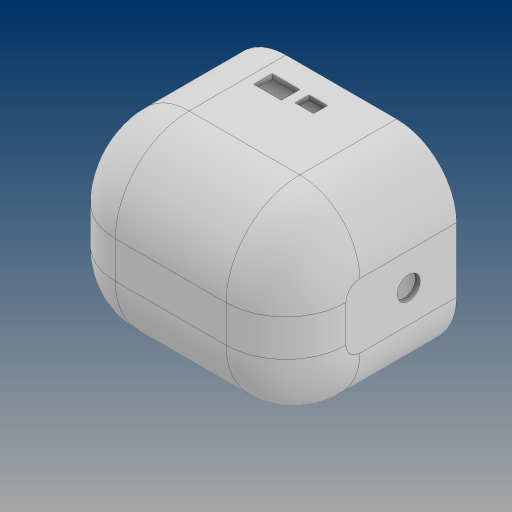
# Autodesk Inventor part: Protosaber Case
Saved by Autodesk Inventor 2023 (Build 270158000, 158)
## iProperties
Created: 2023-05-22
Part Number: Protosaber Case
Material: Generic
Document SubType Name: Modeling
Designer: joosv
Density: 1 g/cm^3
Appearance: Default
Author: joosv
Autodesk Inventor part; units mm, degrees
ref_plane "YZ Plane" through (0, 0, 0) normal (1, 0, 0) x (0, 1, 0)
ref_plane "XZ Plane" through (0, 0, 0) normal (0, 1, 0) x (-1, 0, 0)
ref_plane "XY Plane" through (0, 0, 0) normal (0, 0, 1) x (1, 0, 0)
sketch "Sketch1" plane through (0, 0, 0) normal (0, 0, 1) x (1, 0, 0)
  line L0 (-175, 0) -> (175, 0) projected
  line L1 (0, -140) -> (0, 140) projected
  line L2 (-125, 100) -> (125, 100)
  line L3 (125, 100) -> (125, -100)
  line L4 (125, -100) -> (-125, -100)
  line L5 (-125, -100) -> (-125, 100)
  point P0 (0, 0)
  dimension "d0" = 200
  dimension "d1" = 250
  constraints: 8 end point, 2 parallel, 1 horizontal, 1 perpendicular, 2 other
  measures "d0" distance of L4.end L2.start
  measures "d1" distance of L2.start L2.end
extrude "Extrusion1" add sketch "Sketch1" against normal blind 180
fillet "Fillet5" radius 80 2 edges at (0, -100, 0) (0, 100, 0)
fillet "Fillet6" radius 65 10 edges at (125, 0, 0) (125, 76.5685, -23.4315) (125, 100, -130) (125, -100, -130) (125, -76.5685, -23.4315) (-125, -100, -130) (-125, 0, 0) (-125, 76.5685, -23.4315) (-125, 100, -130) (-125, -76.5685, -23.4315)
shell "Shell1" thickness 5 removed faces 1 at (20, -33.3333, -180)
sketch "Sketch5" plane through (-60, -100, -180) normal (0, -1, 0) x (1, 0, 0)
  line L0 (120, 0) -> (120, 100) projected
  line L1 (70, 96.5308) -> (120, 96.5308)
  line L2 (120, 96.5308) -> (120, 71.5308)
  line L3 (120, 71.5308) -> (70, 71.5308)
  line L4 (70, 71.5308) -> (70, 96.5308)
  point P0 (60, 180)
  dimension "d15" = 25
  dimension "d16" = 50
  constraints: 8 end point, 2 parallel, 1 horizontal, 1 perpendicular, 1 point on line
  measures "d15" distance between parallel lines of L3 L1
  measures "d16" distance between parallel lines of L0 L4
extrude "Extrusion3" cut sketch "Sketch5" against normal blind 24
sketch "Sketch6" plane through (-60, -100, -80) normal (0, -1, 0) x (1, 0, 0)
  circle A0 centre (55, -15.7839) radius 7.5
  line L0 (70, -28.4692) -> (70, -3.4692) projected
  point P0 (60, 80)
  point P1 (70, -15.9692)
  dimension "d19" = 15
  dimension "d20" = 15
  constraints: 1 centre point, 1 midpoint
  measures "d19" diameter of A0
  measures "d20" horizontal distance of point (70, -15.969) A0.centre
extrude "Extrusion4" add sketch "Sketch6" along normal blind 25
sketch "Sketch7" plane through (-60, -100, -80) normal (0, -1, 0) x (1, 0, 0)
  circle A0 centre (95, -60.7349) radius 11
  line L0 (120, -28.4692) -> (120, -100) projected
  point P0 (60, 80)
  dimension "d23" = 25
  dimension "d24" = 22
  constraints: 1 centre point
  measures "d23" distance from line of L0 A0.centre
  measures "d24" diameter of A0
extrude "Extrusion5" add sketch "Sketch7" along normal blind 20
fillet "Fillet7" radius 1.5 1 edges at (-12.5, -125, -95.7839)
fillet "Fillet8" radius 1.5 1 edges at (24, -120, -140.7349)
sketch "Sketch8" plane through (-60, -95, -180) normal (0, 1, 0) x (1, 0, 0)
  line L0 (120, -96.5308) -> (70, -96.5308) projected
  line L1 (70, -96.5308) -> (70, -71.5308) projected
  line L2 (70, -71.5308) -> (120, -71.5308) projected
  line L3 (120, -71.5308) -> (120, 0) projected
  line L4 (0, 0) -> (120, 0) projected
  line L5 (0, 0) -> (0, -100) projected
  line L6 (0, -100) -> (120, -100) projected
  line L7 (120, -100) -> (120, -96.5308) projected
  line L8 (103.331, -9.0858) -> (93.331, -9.0858)
  line L9 (93.331, -9.0858) -> (93.331, -12.0858)
  line L10 (93.331, -12.0858) -> (103.331, -12.0858)
  line L11 (103.331, -12.0858) -> (103.331, -9.0858)
  line L12 (60, -9.0858) -> (50, -9.0858)
  line L13 (50, -9.0858) -> (50, -12.0858)
  line L14 (50, -12.0858) -> (60, -12.0858)
  line L15 (60, -12.0858) -> (60, -9.0858)
  point P0 (60, -180)
  dimension "d29" = 10
  dimension "d30" = 3
  dimension "d31" = 10
  constraints: 16 end point, 4 parallel, 2 horizontal, 2 perpendicular, 2 point on line
  measures "d29" distance of L10.end L9.end
  measures "d30" distance of L9.end L8.end
  measures "d31" distance of L14.end L13.end
extrude "Extrusion6" add sketch "Sketch8" along normal blind 15 contours L11 L10 L9 L8 | L15 L14 L13 L12
sketch "Sketch9" plane through (-10, -95, -167.9142) normal (0, 0, 1) x (1, 0, 0)
  line L0 (0, 0) -> (0, 15) projected
  line L1 (10, 0) -> (10, 15) projected
  line L2 (0, 9.5743) -> (10, 9.5743)
  line L3 (10, 9.5743) -> (10, 15)
  line L4 (10, 15) -> (0, 15)
  line L5 (0, 15) -> (0, 9.5743)
  line L6 (53.331, 15) -> (43.331, 15) projected
  line L7 (43.2725, 9.5743) -> (53.331, 9.5743)
  line L8 (53.331, 9.5743) -> (53.331, 15)
  line L9 (53.331, 15) -> (43.2725, 15)
  line L10 (43.2725, 15) -> (43.2725, 9.5743)
  point P0 (10, 95)
  constraints: 16 end point, 4 parallel, 2 horizontal, 2 perpendicular, 2 point on line
extrude "Extrusion7" add sketch "Sketch9" along normal blind 5
sketch "Sketch10" plane through (125, -35, -180) normal (1, 0, 0) x (0, 0, -1)
  line L0 (0, 0) -> (-100, 0) projected
  line L1 (0, 70) -> (0, 0) projected
  line L2 (-100, 70) -> (0, 70) projected
  arc A0 (-100, 70) -> (-115, 55) centre (-100, 55) ccw projected
  line L3 (-115, 15) -> (-115, 55) projected
  arc A1 (-115, 15) -> (-100, 0) centre (-100, 15) ccw projected
  circle A2 centre (-47.024, 35) radius 12.5
  point P0 (-180, 35)
  dimension "d36" = 25
  constraints: 1 centre point
  measures "d36" diameter of A2
extrude "Extrusion8" cut sketch "Sketch10" against normal blind 25 contours A2
sketch "Sketch11" plane through (-60, 100, -80) normal (0, 1, 0) x (1, 0, 0)
  line L0 (40, 60) -> (10, 60)
  line L1 (10, 60) -> (10, 80)
  line L2 (10, 80) -> (40, 80)
  line L3 (40, 80) -> (40, 60)
  line L4 (0, 0) -> (0, 100) projected
  line L5 (0, 100) -> (120, 100) projected
  point P0 (60, -80)
  point P1 (10, 70)
  dimension "d41" = 30
  dimension "d42" = 20
  dimension "d43" = 10
  dimension "d44" = 20
  constraints: 8 end point, 2 parallel, 1 horizontal, 1 midpoint, 1 perpendicular
  measures "d41" distance of L1.end L2.end
  measures "d42" distance of L0.end L1.end
  measures "d43" distance from line of L4 point (10, 70)
  measures "d44" distance between parallel lines of L5 L2
extrude "Extrusion9" cut sketch "Sketch11" against normal blind 10
sketch "Sketch12" plane through (-60, 100, -80) normal (0, 1, 0) x (1, 0, 0)
  line L0 (70, 65) -> (50, 65)
  line L1 (50, 65) -> (50, 80)
  line L2 (50, 80) -> (70, 80)
  line L3 (70, 80) -> (70, 65)
  line L4 (40, 80) -> (40, 60) projected
  line L5 (0, 100) -> (120, 100) projected
  point P0 (60, -80)
  dimension "d47" = 10
  dimension "d48" = 20
  dimension "d49" = 15
  dimension "d50" = 20
  constraints: 8 end point, 2 parallel, 1 horizontal, 1 perpendicular
  measures "d47" distance between parallel lines of L4 L1
  measures "d48" distance of L0.start L0.end
  measures "d49" distance of L2.end L0.start
  measures "d50" distance between parallel lines of L5 L2
extrude "Extrusion10" cut sketch "Sketch12" against normal blind 10
sketch "Sketch13" plane through (0, 0, -180) normal (0, 0, -1) x (-1, 0, 0)
  arc A0 (-60, 95) -> (-120, 35) centre (-60, 35) ccw projected
  line L0 (-60, 95) -> (60, 95) projected
  arc A1 (120, 35) -> (60, 95) centre (60, 35) ccw projected
  line L1 (120, 35) -> (120, -35) projected
  arc A2 (60, -95) -> (120, -35) centre (60, -35) ccw projected
  line L2 (60, -95) -> (-60, -95) projected
  arc A3 (-120, -35) -> (-60, -95) centre (-60, -35) ccw projected
  line L3 (-120, -35) -> (-120, 35) projected
  arc A4 (125, 35) -> (60, 100) centre (60, 35) ccw projected
  line L4 (60, 100) -> (-60, 100) projected
  arc A5 (-60, 100) -> (-125, 35) centre (-60, 35) ccw projected
  line L5 (-125, 35) -> (-125, -35) projected
  arc A6 (-125, -35) -> (-60, -100) centre (-60, -35) ccw projected
  line L6 (-60, -100) -> (60, -100) projected
  arc A7 (60, -100) -> (125, -35) centre (60, -35) ccw projected
  line L7 (125, -35) -> (125, 35) projected
  line L8 (193.8467, 0) -> (-193.8467, 0) projected
  line L9 (0, -172.6924) -> (0, 161.1543) projected
  point P0 (0, 0)
extrude "Extrusion11" add sketch "Sketch13" along normal blind 5
body "Solid1"
